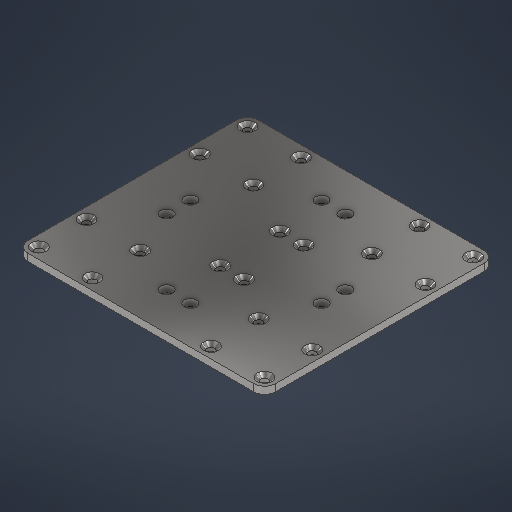
# Autodesk Inventor part: CNC-005-XAxisMount1
Saved by Autodesk Inventor 2026.2 (Build 302298000, 298)
## iProperties
Created: 2026-06-15
Part Number: CNC-005-XAxisMount1
Material: Steel AISI 1008 91 HR
Document SubType Name: Modeling
Designer: Kenji
Density: 7.872 g/cm^3
Appearance: Steel - Polished
Mass: 921.028 g
Surface Area: 548.758 cm^2
Volume: 117.001 cm^3
Author: Kenji
Autodesk Inventor part; units mm, degrees
ref_plane "YZ Plane" through (0, 0, 0) normal (1, 0, 0) x (0, 1, 0)
ref_plane "XZ Plane" through (0, 0, 0) normal (0, 1, 0) x (-1, 0, 0)
ref_plane "XY Plane" through (0, 0, 0) normal (0, 0, 1) x (1, 0, 0)
sketch "Sketch1" plane through (0, 0, 0) normal (0, 1, 0) x (-1, 0, 0)
  circle A0 centre (-12, 20) radius 2.6
  circle A1 centre (4, 20) radius 2.6
  circle A2 centre (4, -20) radius 2.6
  circle A3 centre (-12, -20) radius 2.6
  circle A4 centre (39.75, 38) radius 2.6
  circle A5 centre (39.75, 70) radius 2.6
  circle A6 centre (75.75, 70) radius 2.6
  circle A7 centre (75.75, 38) radius 2.6
  circle A8 centre (39.75, -38) radius 2.6
  circle A9 centre (75.75, -38) radius 2.6
  circle A10 centre (75.75, -70) radius 2.6
  circle A11 centre (39.75, -70) radius 2.6
  circle A12 centre (-39.75, 38) radius 2.6
  circle A13 centre (-39.75, 70) radius 2.6
  circle A14 centre (-75.75, 70) radius 2.6
  circle A15 centre (-75.75, 38) radius 2.6
  circle A16 centre (-39.75, -38) radius 2.6
  circle A17 centre (-39.75, -70) radius 2.6
  circle A18 centre (-75.75, -38) radius 2.6
  circle A19 centre (-75.75, -70) radius 2.6
  line L0 (-78.35, 8) -> (78.35, 8) construction
  line L1 (78.35, 8) -> (78.35, -8) construction
  line L2 (78.35, -8) -> (-78.35, -8) construction
  line L3 (-78.35, -8) -> (-78.35, 8) construction
  line L4 (8, 72.6) -> (-8, 72.6) construction
  line L5 (-8, 72.6) -> (-8, -72.6) construction
  line L6 (-8, -72.6) -> (8, -72.6) construction
  line L7 (8, -72.6) -> (8, 72.6) construction
  circle A20 centre (8, 52) radius 4.1
  line L8 (0, 0) -> (0, 72.6) construction
  line L9 (0, 0) -> (78.35, 0) construction
  circle A21 centre (52, 8) radius 4.1
  circle A22 centre (52, -8) radius 4.1
  circle A23 centre (8, -52) radius 4.1
  circle A24 centre (-8, 52) radius 4.1
  circle A25 centre (-52, 8) radius 4.1
  circle A26 centre (-52, -8) radius 4.1
  circle A27 centre (-8, -52) radius 4.1
  circle A28 centre (75.75, 70) radius 7.3625 construction
  circle A29 centre (75.75, -70) radius 7.3625 construction
  circle A30 centre (-75.75, -70) radius 7.3625 construction
  circle A31 centre (-75.75, 70) radius 7.3625 construction
  line L10 (83.1125, 70) -> (83.1125, -70)
  line L11 (75.75, -77.3625) -> (-75.75, -77.3625)
  line L12 (-83.1125, -70) -> (-83.1125, 70)
  line L13 (-75.75, 77.3625) -> (75.75, 77.3625)
  arc A32 (75.75, -77.3625) -> (83.1125, -70) centre (75.75, -70) ccw
  arc A33 (83.1125, 70) -> (75.75, 77.3625) centre (75.75, 70) ccw
  arc A34 (-75.75, 77.3625) -> (-83.1125, 70) centre (-75.75, 70) ccw
  arc A35 (-83.1125, -70) -> (-75.75, -77.3625) centre (-75.75, -70) ccw
  dimension "d0" = 5.2
  dimension "d1" = 12
  dimension "d2" = 20
  dimension "d3" = 16
  dimension "d4" = 20
  dimension "d5" = 18
  dimension "d6" = 35.75
  dimension "d7" = 32
  dimension "d8" = 36
  dimension "d9" = 18
  dimension "d10" = 32
  dimension "d11" = 27.75
  dimension "d12" = 36
  dimension "d13" = 16
  dimension "d14" = 8
  dimension "d15" = 8
  dimension "d16" = 8.2
  dimension "d18" = 18
  dimension "d20" = 31.75
  dimension "d22" = 30
  dimension "d26" = 4.7625
  dimension "d38" = 8
  dimension "d39" = 8
  dimension "d40" = 8
  dimension "d41" = 52
  dimension "d42" = 52
  dimension "d44" = 52
  constraints: 36 centre point, 28 end point, 28 equal radius, 16 point on circle, 16 vertical alignment, 14 horizontal alignment, 13 tangent, 4 coincident, 4 parallel, 4 perpendicular, 4 symmetric about line, 2 horizontal, 2 midpoint, 4 other
  measures "d0" diameter of A0
  measures "d1" horizontal distance of A0.centre point (0, 0)
  measures "d2" vertical distance of point (0, 0) A0.centre
  measures "d3" distance of A0.centre A1.centre
  measures "d4" vertical distance of A3.centre point (0, 0)
  measures "d5" vertical distance of A4.centre A1.centre
  measures "d6" horizontal distance of A1.centre A4.centre
  measures "d7" distance of A5.centre A4.centre
  measures "d8" distance of A5.centre A6.centre
  measures "d9" vertical distance of A2.centre A8.centre
  measures "d10" distance of A11.centre A8.centre
  measures "d11" horizontal distance of A12.centre A0.centre
  measures "d12" distance of A15.centre A12.centre
  measures "d13" distance of L0.end L1.end
  measures "d14" distance from line of L8.start L0
  measures "d15" distance from line of L5 point (0, 0)
  measures "d16" diameter of A20
  measures "d18" vertical distance of A20.centre A5.centre
  measures "d20" horizontal distance of A20.centre A5.centre
  measures "d22" distance from line of L0 A7.centre
  measures "d26" radial gap between concentric circles of A28 A6
  measures "d38" distance from line of A21.centre L9
  measures "d39" distance from line of L8 A20.centre
  measures "d40" distance from line of A22.centre L9
  measures "d41" vertical distance of A20.centre point (0, 0)
  measures "d42" horizontal distance of point (0, 0) A21.centre
  measures "d44" vertical distance of A23.centre point (0, 0)
extrude "Extrusion1" add sketch "Sketch1" along normal blind 4.7625
sketch "Sketch2" plane through (0, 4.7625, 0) normal (0, 1, 0) x (1, 0, 0)
  line L0 (83.1125, -70) -> (83.1125, 70) projected
  arc A0 (83.1125, 70) -> (75.75, 77.3625) centre (75.75, 70) ccw projected
  line L1 (75.75, 77.3625) -> (-75.75, 77.3625) projected
  arc A1 (-75.75, 77.3625) -> (-83.1125, 70) centre (-75.75, 70) ccw projected
  line L2 (-83.1125, 70) -> (-83.1125, -70) projected
  arc A2 (-83.1125, -70) -> (-75.75, -77.3625) centre (-75.75, -70) ccw projected
  line L3 (-75.75, -77.3625) -> (75.75, -77.3625) projected
  arc A3 (75.75, -77.3625) -> (83.1125, -70) centre (75.75, -70) ccw projected
  circle A4 centre (8, 52) radius 4.1 projected
  circle A5 centre (8, -52) radius 4.1 projected
  circle A6 centre (-8, 52) radius 4.1 projected
  circle A7 centre (-52, -8) radius 4.1 projected
  circle A8 centre (75.75, 38) radius 2.6 projected
  circle A9 centre (39.75, 38) radius 2.6 projected
  circle A10 centre (39.75, -70) radius 2.6 projected
  circle A11 centre (-39.75, 70) radius 2.6 projected
  circle A12 centre (-39.75, 38) radius 2.6 projected
  circle A13 centre (-75.75, -38) radius 2.6 projected
  circle A14 centre (-39.75, -70) radius 2.6 projected
  circle A15 centre (-39.75, -38) radius 2.6 projected
  circle A16 centre (12, 20) radius 2.6 projected
  circle A17 centre (-4, 20) radius 2.6 projected
  circle A18 centre (-4, -20) radius 2.6 projected
  circle A19 centre (12, -20) radius 2.6 projected
  circle A20 centre (-75.75, 38) radius 2.6 projected
  circle A21 centre (39.75, -38) radius 2.6 projected
  circle A22 centre (75.75, -38) radius 2.6 projected
  circle A23 centre (39.75, 70) radius 2.6 projected
  circle A24 centre (-8, -52) radius 4.1 projected
  circle A25 centre (-52, 8) radius 4.1 projected
  circle A26 centre (52, -8) radius 4.1 projected
  circle A27 centre (52, 8) radius 4.1 projected
  circle A28 centre (75.75, 70) radius 2.6 projected
  circle A29 centre (75.75, -70) radius 2.6 projected
  circle A30 centre (-75.75, 70) radius 2.6 projected
  circle A31 centre (-75.75, -70) radius 2.6 projected
  point P0 (0, 0)
hole "Hole1" at (-75.75, 4.7625, 38) at (-75.75, 4.7625, 70) at (-39.75, 4.7625, 70) at (-39.75, 4.7625, 38) at (-75.75, 4.7625, -38) at (-75.75, 4.7625, -70) at (-39.75, 4.7625, -70) at (-39.75, 4.7625, -38) at (-4, 4.7625, -20) at (12, 4.7625, -20) at (12, 4.7625, 20) at (-4, 4.7625, 20) at (39.75, 4.7625, 38) at (75.75, 4.7625, 38) at (39.75, 4.7625, 70) at (75.75, 4.7625, 70) at (75.75, 4.7625, -38) at (39.75, 4.7625, -38) at (39.75, 4.7625, -70) at (75.75, 4.7625, -70) direction (0, -1, 0) diameter 4.019 end through all countersink diameter 10 countersink angle 90 thread size "M5" standard "Din Taper"
equation "\"d4\" = d2"
equation "\"d9\" = d5"
equation "\"d10\" = d7"
equation "\"d12\" = d8"
equation "\"d15\" = d14"
equation "\"d18\" = 0.5 * d8"
equation "\"d38\" = d39"
equation "\"d40\" = d38"
equation "\"d42\" = d41"
equation "\"d44\" = d41"
body "Solid1"
